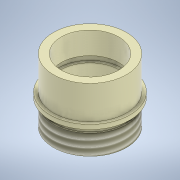
# Autodesk Inventor part: Heated tube-top connector
Saved by Autodesk Inventor 2020 (Build 240168000, 168)
## iProperties
Created: 2020-06-19
Part Number: Heated tube-top connector
Material: Polypropylene
Document SubType Name: Modeling
Designer: Juan
Density: 0.899 g/cm^3
Appearance: Smooth - Ash
Author: Juan
Autodesk Inventor part; units mm, degrees
ref_plane "YZ Plane" through (0, 0, 0) normal (1, 0, 0) x (0, 1, 0)
ref_plane "XZ Plane" through (0, 0, 0) normal (0, 1, 0) x (-1, 0, 0)
ref_plane "XY Plane" through (0, 0, 0) normal (0, 0, 1) x (1, 0, 0)
sketch "Sketch2" plane through (0, 0, 0) normal (0, 0, 1) x (1, 0, 0)
  line L0 (0, 0) -> (0, 30)
  line L1 (0, 30) -> (-16.5, 30)
  line L2 (0, 0) -> (-13, 0)
  line L3 (-13, 0) -> (-16.5, 0)
  line L4 (-13, 30) -> (-13, 20)
  line L5 (-13, 20) -> (-14.35, 20)
  line L6 (-14.35, 20) -> (-14.35, 17.2)
  line L7 (-14.35, 17.2) -> (-13, 17.2)
  line L8 (-13, 17.2) -> (-13, 0)
  line L9 (-16.5, 13) -> (-15.8, 13)
  line L10 (-15.8, 13) -> (-15.8, 10.5)
  line L11 (-15.8, 10.5) -> (-16.5, 10.5)
  line L12 (-16.5, 30) -> (-16.5, 15)
  line L13 (-16.5, 15) -> (-18, 15)
  line L14 (-18, 15) -> (-18, 13)
  line L15 (-18, 13) -> (-16.5, 13)
  line L16 (-16.5, 10.5) -> (-16.5, 1.5)
  line L17 (-16.5, 1.5) -> (-13, 1.5)
  dimension "d4" = 30
  dimension "d5" = 16.5
  dimension "d6" = 13
  dimension "d7" = 10
  dimension "d8" = 1.35
  dimension "d9" = 2.8
  dimension "d13" = 17
  dimension "d14" = 0.7
  dimension "d15" = 2.5
  dimension "d18" = 15
  dimension "d19" = 1.5
  dimension "d20" = 10.5
  dimension "d21" = 9
  constraints: 36 end point, 8 perpendicular, 4 vertical, 3 point on line, 2 collinear, 1 horizontal, 1 parallel
  measures "d4" distance of L0.start L0.end
  measures "d5" distance of L0.end L1.end
  measures "d6" distance of L0.start L2.end
  measures "d7" distance of L4.start L4.end
  measures "d8" distance of L4.end L5.end
  measures "d9" distance of L5.end L6.end
  measures "d13" distance of L1.end L9.start
  measures "d14" distance of L9.start L9.end
  measures "d15" distance of L9.end L10.end
  measures "d18" distance of L1.end L12.end
  measures "d19" distance of L12.end L13.end
  measures "d20" distance of L11.end L3.end
  measures "d21" distance of L11.end L16.end
revolve "Revolution1" add sketch "Sketch2" angle 360 about axis through (0, 0, 0) along (0, 1, 0) contours L4 L5 L6 L7 L8 L17 L16 L11 L10 L9 L15 L14 L13 L12 L1
thread "Thread3" size "M33x3" class "6g" standard "ANSI Metric M Profile" full length
body "Solid2"
